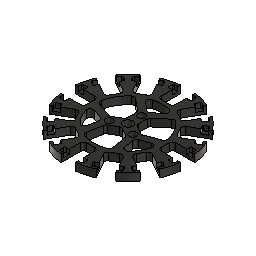
omni_wheel (Autodesk Fusion 360 archive; units mm, degrees)
design "omni_inside_world"
Autodesk Fusion 360 part; units mm, degrees
(part 1 of 2)
sketch "スケッチ1" plane through (0, 0, 0) normal (0, 0, 1) x (1, 0, 0)
  circle A0 centre (0, 0) radius 27.5
  line L0 (0, 0) -> (0, 27.5)
  line L1 (0, 27.5) -> (0, 17)
  line L2 (0, 17) -> (3.3, 17)
  line L3 (3.3, 17) -> (3.3, 27.3013)
  line L4 (3.3, 17) -> (-3.3, 17)
  line L5 (-3.3, 17) -> (-3.3, 27.5)
  line L6 (-3.3, 27.5) -> (3.3, 27.5)
  line L7 (3.3, 27.5) -> (3.3, 17)
  line L8 (-11.3579, 13.0724) -> (-16.6079, 22.1657)
  line L9 (-5.6421, 16.3724) -> (-11.3579, 13.0724)
  line L10 (-5.6421, 16.3724) -> (-10.7928, 25.2936)
  line L11 (-16.6079, 22.1657) -> (-10.8921, 25.4657)
  line L12 (-8.5, 14.7224) -> (-5.6421, 16.3724)
  line L13 (-16.3724, 5.6421) -> (-25.4657, 10.8921)
  line L14 (-13.0724, 11.3579) -> (-16.3724, 5.6421)
  line L15 (-13.0724, 11.3579) -> (-21.9936, 16.5085)
  line L16 (-25.4657, 10.8921) -> (-22.1657, 16.6079)
  line L17 (-14.7224, 8.5) -> (-13.0724, 11.3579)
  line L18 (-17, -3.3) -> (-27.5, -3.3)
  line L19 (-17, 3.3) -> (-17, -3.3)
  line L20 (-17, 3.3) -> (-27.3013, 3.3)
  line L21 (-27.5, -3.3) -> (-27.5, 3.3)
  line L22 (-17, 0) -> (-17, 3.3)
  line L23 (-13.0724, -11.3579) -> (-22.1657, -16.6079)
  line L24 (-16.3724, -5.6421) -> (-13.0724, -11.3579)
  line L25 (-16.3724, -5.6421) -> (-25.2936, -10.7928)
  line L26 (-22.1657, -16.6079) -> (-25.4657, -10.8921)
  line L27 (-14.7224, -8.5) -> (-16.3724, -5.6421)
  line L28 (-5.6421, -16.3724) -> (-10.8921, -25.4657)
  line L29 (-11.3579, -13.0724) -> (-5.6421, -16.3724)
  line L30 (-11.3579, -13.0724) -> (-16.5085, -21.9936)
  line L31 (-10.8921, -25.4657) -> (-16.6079, -22.1657)
  line L32 (-8.5, -14.7224) -> (-11.3579, -13.0724)
  line L33 (3.3, -17) -> (3.3, -27.5)
  line L34 (-3.3, -17) -> (3.3, -17)
  line L35 (-3.3, -17) -> (-3.3, -27.3013)
  line L36 (3.3, -27.5) -> (-3.3, -27.5)
  line L37 (0, -17) -> (-3.3, -17)
  line L38 (11.3579, -13.0724) -> (16.6079, -22.1657)
  line L39 (5.6421, -16.3724) -> (11.3579, -13.0724)
  line L40 (5.6421, -16.3724) -> (10.7928, -25.2936)
  line L41 (16.6079, -22.1657) -> (10.8921, -25.4657)
  line L42 (8.5, -14.7224) -> (5.6421, -16.3724)
  line L43 (16.3724, -5.6421) -> (25.4657, -10.8921)
  line L44 (13.0724, -11.3579) -> (16.3724, -5.6421)
  line L45 (13.0724, -11.3579) -> (21.9936, -16.5085)
  line L46 (25.4657, -10.8921) -> (22.1657, -16.6079)
  line L47 (14.7224, -8.5) -> (13.0724, -11.3579)
  line L48 (17, 3.3) -> (27.5, 3.3)
  line L49 (17, -3.3) -> (17, 3.3)
  line L50 (17, -3.3) -> (27.3013, -3.3)
  line L51 (27.5, 3.3) -> (27.5, -3.3)
  line L52 (17, 0) -> (17, -3.3)
  line L53 (13.0724, 11.3579) -> (22.1657, 16.6079)
  line L54 (16.3724, 5.6421) -> (13.0724, 11.3579)
  line L55 (16.3724, 5.6421) -> (25.2936, 10.7928)
  line L56 (22.1657, 16.6079) -> (25.4657, 10.8921)
  line L57 (14.7224, 8.5) -> (16.3724, 5.6421)
  line L58 (5.6421, 16.3724) -> (10.8921, 25.4657)
  line L59 (11.3579, 13.0724) -> (5.6421, 16.3724)
  line L60 (11.3579, 13.0724) -> (16.5085, 21.9936)
  line L61 (10.8921, 25.4657) -> (16.6079, 22.1657)
  line L62 (8.5, 14.7224) -> (11.3579, 13.0724)
  line L63 (0, 17) -> (0, 15.5)
  circle A1 centre (0, 0) radius 15.5
  circle A2 centre (0, 0) radius 2.1
  line L64 (0, 2.1) -> (2.5, 2.1)
  line L65 (2.5, 2.1) -> (2.5, 15.2971)
  line L66 (2.5, 2.1) -> (-2.5, 2.1)
  line L67 (-2.5, 2.1) -> (-2.5, 15.2971)
  line L68 (-2.5, 15.2971) -> (2.5, 15.2971)
  line L69 (2.5, 15.2971) -> (2.5, 2.1)
  line L70 (-2.5, 2.1) -> (2.5, 2.1)
  line L71 (2.5, 2.1) -> (2.5, 0)
  line L72 (2.5, 0) -> (-2.5, 0)
  line L73 (-2.5, 0) -> (-2.5, 2.1)
  line L74 (1.25, -2.1651) -> (-0.5687, -3.2151)
  line L75 (-0.5687, -3.2151) -> (-11.9976, -9.8136)
  line L76 (-3.0687, 1.1151) -> (-1.25, 2.1651)
  line L77 (-3.0687, 1.1151) -> (-14.4976, -5.4835)
  line L78 (-1.25, 2.1651) -> (1.25, -2.1651)
  line L79 (1.25, 2.1651) -> (3.0687, 1.1151)
  line L80 (3.0687, 1.1151) -> (14.4976, -5.4835)
  line L81 (0.5687, -3.2151) -> (-1.25, -2.1651)
  line L82 (0.5687, -3.2151) -> (11.9976, -9.8136)
  line L83 (-1.25, -2.1651) -> (1.25, 2.1651)
  line L84 (0, 0) -> (0, 6.8)
  line L85 (0, 6.8) -> (-2.5, 6.8)
  line L86 (0, 6.8) -> (2.5, 6.8)
  line L87 (0, 6.8) -> (7.8674, 13.3549)
  line L88 (0, 6.8) -> (9.0795, 6.8) construction
  line L89 (0, 6.8) -> (0.9602, 5.6476)
  line L90 (0.9602, 5.6476) -> (9.1755, 12.4924)
  line L91 (0, 6.8) -> (-0.9602, 7.9524)
  line L92 (-0.9602, 7.9524) -> (6.4251, 14.1056)
  line L93 (0.9602, 7.9524) -> (-6.4251, 14.1056)
  line L94 (-0.9602, 5.6476) -> (-9.1755, 12.4924)
  line L95 (0, 6.8) -> (-7.8674, 13.3549)
  line L96 (0, 6.8) -> (-0.9602, 5.6476)
  line L97 (0, 6.8) -> (0.9602, 7.9524)
  line L98 (-7.3671, -3.1447) -> (-9.0033, -12.6171)
  line L99 (-5.889, -3.4) -> (-7.632, -13.4909)
  line L100 (-4.4109, -3.6553) -> (-6.2309, -14.1924)
  line L101 (-6.4069, -4.8077) -> (-15.4284, -1.4885)
  line L102 (-5.889, -3.4) -> (-15.4994, 0.136)
  line L103 (-5.371, -1.9923) -> (-15.4065, 1.7001)
  line L104 (-5.889, -3.4) -> (-5.371, -1.9923)
  line L105 (-5.889, -3.4) -> (-4.4109, -3.6553)
  line L106 (-5.889, -3.4) -> (-6.4069, -4.8077)
  line L107 (-5.889, -3.4) -> (-7.3671, -3.1447)
  line L108 (6.4069, -4.8077) -> (15.4284, -1.4885)
  line L109 (5.889, -3.4) -> (15.4994, 0.136)
  line L110 (5.371, -1.9923) -> (15.4065, 1.7001)
  line L111 (7.3671, -3.1447) -> (9.0033, -12.6171)
  line L112 (5.889, -3.4) -> (7.632, -13.4909)
  line L113 (4.4109, -3.6553) -> (6.2309, -14.1924)
  line L114 (5.889, -3.4) -> (4.4109, -3.6553)
  line L115 (5.889, -3.4) -> (5.371, -1.9923)
  line L116 (5.889, -3.4) -> (7.3671, -3.1447)
  line L117 (5.889, -3.4) -> (6.4069, -4.8077)
  dimension "d1" = 55
  dimension "d2" = 10.5
  dimension "d3" = 3.3
  dimension "d4" = 6.6
  dimension "d5" = 10.5
  dimension "d7" = 360
  dimension "d8" = 1.5
  dimension "d9" = 4.2
  dimension "d10" = 2.5
  dimension "d11" = 5
  dimension "d12" = 5
  dimension "d13" = 2.1
  dimension "d15" = 360
  dimension "d16" = 6.8
  dimension "d17" = 39.8
  dimension "d18" = 1.5
  dimension "d19" = 1.5
  dimension "d56" = 360
  constraint coincident A0.centre L0.start
  constraint coincident A0 L0.end
  constraint vertical L0
  constraint parallel L0 L1
  constraint perpendicular L0 L2
  constraint coincident A0 L3.end
  constraint perpendicular L2 L3
  constraint horizontal L4
  constraint vertical L5
  constraint horizontal L6
  constraint vertical L7
  constraint perpendicular L2 L63
  constraint concentric A0 A1
  constraint coincident L63.end A1
  constraint coincident L0 L64.start
  constraint coincident A2 L64.start
  constraint perpendicular L0 L64
  constraint coincident A1 L65.end
  constraint perpendicular L64 L65
  constraint horizontal L66
  constraint vertical L67
  constraint horizontal L68
  constraint vertical L69
  constraint coincident A1 L67.end
  constraint horizontal L70
  constraint vertical L71
  constraint horizontal L72
  constraint vertical L73
  constraint parallel L0 L84
  constraint coincident L67 L85.end
  constraint perpendicular L67 L85
  constraint coincident L69 L86.end
  constraint perpendicular L69 L86
  constraint horizontal L88
  constraint coincident A1 L87.end
  constraint perpendicular L87 L89
  constraint coincident A1 L90.end
  constraint perpendicular L89 L90
  constraint perpendicular L87 L91
  constraint coincident A1 L92.end
  constraint perpendicular L91 L92
  constraint symmetric L0 L84.end L85.start
  constraint symmetric L0 L87.end L95.end
  constraint symmetric L0 L89.end L94.start
  constraint symmetric L0 L90.end L94.end
  constraint symmetric L0 L91.end L93.start
  constraint symmetric L0 L92.end L93.end
  measures "d1" diameter of A0
  measures "d2" distance of L0.end L1.end
  measures "d3" distance of L1.end L2.end
  measures "d4" distance of L2.end L4.end
  measures "d5" distance of L2.end L6.end
  measures "d8" distance of L1.end L63.end
  measures "d9" diameter of A2
  measures "d10" distance of L64.start L64.end
  measures "d11" distance of L64.end L66.end
  measures "d12" distance of L66.end L64.end
  measures "d13" distance of L66.end L72.end
  measures "d16" distance of A0.centre L84.end
  measures "d17" angle of L87 L88
  measures "d18" distance of L84.end L89.end
  measures "d19" distance of L84.end L91.end
extrude "押し出し1" add sketch "スケッチ1" along normal blind 1.5 contours A0 L2 L3 L4 L5 L7 L8 L9 L10 L12 L13 L14 L15 L17 L18 L19 L20 L22 L23 L24 L25 L27 L28 L29 L30 L32 L33 L34 L35 L37 L38 L39 L40 L42 L43 L44 L45 L47 L48 L49 L50 L52 L53 L54 L55 L57 L58 L59 L60 L62 | L0 L66 L67 L70 L76 L78 L84 L85 L94 L96 | A2 L64 L66 L70 L83 | L0 L64 L65 L66 L69 L70 L79 L83 L84 L86 L89 L90 | A2 L66 L70 L78 | A2 L71 L72 L74 L78 L79 L80 L81 L82 L110 L113 L114 L115 | A2 L64 L66 L70 L71 L72 L79 L83 | A2 L66 L70 L72 L73 L76 L78 | A2 L72 L73 L74 L75 L76 L77 L81 L83 L100 L103 L104 L105 | A2 L74 L78 L81 L83 | L0 L91 L92 | L85 L94 L96 | L65 L69 L86 L87 L90 | L65 L69 L87 L92 L93 L97 | L86 L89 L90 | L67 L91 L92 L93 L95 | L67 L85 L94 L95 | L0 L93 L97 | L64 L66 L70 L79 L83 | L66 L70 L76 L78 | L67 L85 L94 | L65 L69 L86 L90 | A1 L65 L69 L87 L90 | A1 L65 L69 L87 L92 | A1 L67 L93 L95 | A1 L67 L94 L95 | L64 L66 L70 L71 L79 | L66 L70 L73 L76 | A1 L80 L109 L110 | L80 L109 L110 L115 | L77 L102 L103 L104 | A1 L77 L102 L103 | A1 L75 L99 L100 | L75 L99 L100 L105 | L82 L112 L113 L114 | A1 L82 L112 L113 | A1 L80 L108 L109 | L80 L108 L109 L111 L116 | L77 L98 L101 L102 L107 | A1 L77 L101 L102 | A1 L75 L98 L99 | L75 L98 L99 L101 L106 | L82 L108 L111 L112 L117 | A1 L82 L111 L112 | L108 L111 L116 L117 | L98 L101 L106 L107
sketch "スケッチ2" plane through (0, 0, 1.5) normal (0, 0, 1) x (-1, 0, 0)
  line L0 (-5.6421, -16.3724) -> (-10.7928, -25.2936)
  arc A0 (-10.7928, -25.2936) -> (-3.3, -27.3013) centre (0, 0) ccw
  line L1 (-3.3, -27.3013) -> (-3.3, -17)
  line L2 (-3.3, -17) -> (3.3, -17)
  line L3 (3.3, -17) -> (3.3, -27.3013)
  arc A1 (3.3, -27.3013) -> (10.7928, -25.2936) centre (0, 0) ccw
  line L4 (10.7928, -25.2936) -> (5.6421, -16.3724)
  line L5 (5.6421, -16.3724) -> (11.3579, -13.0724)
  line L6 (11.3579, -13.0724) -> (16.5085, -21.9936)
  arc A2 (16.5085, -21.9936) -> (21.9936, -16.5085) centre (0, 0) ccw
  line L7 (21.9936, -16.5085) -> (13.0724, -11.3579)
  line L8 (13.0724, -11.3579) -> (16.3724, -5.6421)
  line L9 (16.3724, -5.6421) -> (25.2936, -10.7928)
  arc A3 (25.2936, -10.7928) -> (27.3013, -3.3) centre (0, 0) ccw
  line L10 (27.3013, -3.3) -> (17, -3.3)
  line L11 (17, -3.3) -> (17, 3.3)
  line L12 (17, 3.3) -> (27.3013, 3.3)
  arc A4 (27.3013, 3.3) -> (25.2936, 10.7928) centre (0, 0) ccw
  line L13 (25.2936, 10.7928) -> (16.3724, 5.6421)
  line L14 (16.3724, 5.6421) -> (13.0724, 11.3579)
  line L15 (13.0724, 11.3579) -> (21.9936, 16.5085)
  arc A5 (21.9936, 16.5085) -> (16.5085, 21.9936) centre (0, 0) ccw
  line L16 (16.5085, 21.9936) -> (11.3579, 13.0724)
  line L17 (11.3579, 13.0724) -> (5.6421, 16.3724)
  line L18 (5.6421, 16.3724) -> (10.7928, 25.2936)
  arc A6 (10.7928, 25.2936) -> (3.3, 27.3013) centre (0, 0) ccw
  line L19 (3.3, 27.3013) -> (3.3, 17)
  line L20 (3.3, 17) -> (-3.3, 17)
  line L21 (-3.3, 17) -> (-3.3, 27.3013)
  arc A7 (-3.3, 27.3013) -> (-10.7928, 25.2936) centre (0, 0) ccw
  line L22 (-10.7928, 25.2936) -> (-5.6421, 16.3724)
  line L23 (-5.6421, 16.3724) -> (-11.3579, 13.0724)
  line L24 (-11.3579, 13.0724) -> (-16.5085, 21.9936)
  arc A8 (-16.5085, 21.9936) -> (-21.9936, 16.5085) centre (0, 0) ccw
  line L25 (-21.9936, 16.5085) -> (-13.0724, 11.3579)
  line L26 (-13.0724, 11.3579) -> (-16.3724, 5.6421)
  line L27 (-16.3724, 5.6421) -> (-25.2936, 10.7928)
  arc A9 (-25.2936, 10.7928) -> (-27.3013, 3.3) centre (0, 0) ccw
  line L28 (-27.3013, 3.3) -> (-17, 3.3)
  line L29 (-17, 3.3) -> (-17, -3.3)
  line L30 (-17, -3.3) -> (-27.3013, -3.3)
  arc A10 (-27.3013, -3.3) -> (-25.2936, -10.7928) centre (0, 0) ccw
  line L31 (-25.2936, -10.7928) -> (-16.3724, -5.6421)
  line L32 (-16.3724, -5.6421) -> (-13.0724, -11.3579)
  line L33 (-13.0724, -11.3579) -> (-21.9936, -16.5085)
  arc A11 (-21.9936, -16.5085) -> (-16.5085, -21.9936) centre (0, 0) ccw
  line L34 (-16.5085, -21.9936) -> (-11.3579, -13.0724)
  line L35 (-11.3579, -13.0724) -> (-5.6421, -16.3724)
  line L36 (0, 0) -> (0, -6.25)
  circle A12 centre (0, -6.25) radius 2.5
  circle A13 centre (0, -6.25) radius 1.65
  circle A14 centre (5.4127, 3.125) radius 2.5
  circle A15 centre (5.4127, 3.125) radius 1.65
  circle A16 centre (-5.4127, 3.125) radius 2.5
  circle A17 centre (-5.4127, 3.125) radius 1.65
  line L37 (4.752, 5.6303) -> (0, 2.8868)
  line L38 (0, 2.8868) -> (-4.752, 5.6303)
  line L39 (-4.752, 5.6303) -> (-6.2309, 14.1924)
  arc A18 (6.2309, 14.1924) -> (-6.2309, 14.1924) centre (0, 0) ccw
  line L40 (6.2309, 14.1924) -> (4.752, 5.6303)
  circle A19 centre (0, 0) radius 2.1
  arc A20 (15.4284, 1.4885) -> (9.0033, 12.6171) centre (0, 0) ccw
  line L41 (15.4284, 1.4885) -> (7.5798, 4.3762)
  line L42 (7.5798, 4.3762) -> (9.0033, 12.6171)
  line L43 (2.5, -6.9305) -> (2.5, -1.4434)
  line L44 (2.5, -1.4434) -> (7.252, 1.3002)
  line L45 (7.252, 1.3002) -> (15.4065, -1.7001)
  arc A21 (9.1755, -12.4924) -> (15.4065, -1.7001) centre (0, 0) ccw
  line L46 (9.1755, -12.4924) -> (2.5, -6.9305)
  arc A22 (-9.0033, 12.6171) -> (-15.4284, 1.4885) centre (0, 0) ccw
  line L47 (-9.0033, 12.6171) -> (-7.5798, 4.3762)
  line L48 (-7.5798, 4.3762) -> (-15.4284, 1.4885)
  line L49 (-6.4251, -14.1056) -> (0, -8.7524)
  line L50 (0, -8.7524) -> (6.4251, -14.1056)
  arc A23 (-6.4251, -14.1056) -> (6.4251, -14.1056) centre (0, 0) ccw
  line L51 (-2.5, -6.9305) -> (-9.1755, -12.4924)
  arc A24 (-15.4065, -1.7001) -> (-9.1755, -12.4924) centre (0, 0) ccw
  line L52 (-15.4065, -1.7001) -> (-7.252, 1.3002)
  line L53 (-7.252, 1.3002) -> (-2.5, -1.4434)
  line L54 (-2.5, -1.4434) -> (-2.5, -6.9305)
  dimension "d25" = 6.25
  dimension "d26" = 5
  dimension "d27" = 3.3
  dimension "d29" = 360
  constraint coincident A0.centre A1.centre
  constraint vertical L36
  constraint coincident L36.end A12.centre
  constraint concentric A12 A13
  measures "d25" distance of A0.centre L36.end
  measures "d26" diameter of A12
  measures "d27" diameter of A13
extrude "押し出し2" cut sketch "スケッチ2" against normal blind 1.5 contours A13 | A15 | A17
sketch "スケッチ3" plane through (0, 0, 1.5) normal (0, 0, 1) x (-1, 0, 0)
  line L0 (-5.6421, -16.3724) -> (-10.7928, -25.2936)
  arc A0 (-10.7928, -25.2936) -> (-3.3, -27.3013) centre (0, 0) ccw
  line L1 (-3.3, -27.3013) -> (-3.3, -17)
  line L2 (-3.3, -17) -> (3.3, -17)
  line L3 (3.3, -17) -> (3.3, -27.3013)
  arc A1 (3.3, -27.3013) -> (10.7928, -25.2936) centre (0, 0) ccw
  line L4 (10.7928, -25.2936) -> (5.6421, -16.3724)
  line L5 (5.6421, -16.3724) -> (11.3579, -13.0724)
  line L6 (11.3579, -13.0724) -> (16.5085, -21.9936)
  arc A2 (16.5085, -21.9936) -> (21.9936, -16.5085) centre (0, 0) ccw
  line L7 (21.9936, -16.5085) -> (13.0724, -11.3579)
  line L8 (13.0724, -11.3579) -> (16.3724, -5.6421)
  line L9 (16.3724, -5.6421) -> (25.2936, -10.7928)
  arc A3 (25.2936, -10.7928) -> (27.3013, -3.3) centre (0, 0) ccw
  line L10 (27.3013, -3.3) -> (17, -3.3)
  line L11 (17, -3.3) -> (17, 3.3)
  line L12 (17, 3.3) -> (27.3013, 3.3)
  arc A4 (27.3013, 3.3) -> (25.2936, 10.7928) centre (0, 0) ccw
  line L13 (25.2936, 10.7928) -> (16.3724, 5.6421)
  line L14 (16.3724, 5.6421) -> (13.0724, 11.3579)
  line L15 (13.0724, 11.3579) -> (21.9936, 16.5085)
  arc A5 (21.9936, 16.5085) -> (16.5085, 21.9936) centre (0, 0) ccw
  line L16 (16.5085, 21.9936) -> (11.3579, 13.0724)
  line L17 (11.3579, 13.0724) -> (5.6421, 16.3724)
  line L18 (5.6421, 16.3724) -> (10.7928, 25.2936)
  arc A6 (10.7928, 25.2936) -> (3.3, 27.3013) centre (0, 0) ccw
  line L19 (3.3, 27.3013) -> (3.3, 17)
  line L20 (3.3, 17) -> (-3.3, 17)
  line L21 (-3.3, 17) -> (-3.3, 27.3013)
  arc A7 (-3.3, 27.3013) -> (-10.7928, 25.2936) centre (0, 0) ccw
  line L22 (-10.7928, 25.2936) -> (-5.6421, 16.3724)
  line L23 (-5.6421, 16.3724) -> (-11.3579, 13.0724)
  line L24 (-11.3579, 13.0724) -> (-16.5085, 21.9936)
  arc A8 (-16.5085, 21.9936) -> (-21.9936, 16.5085) centre (0, 0) ccw
  line L25 (-21.9936, 16.5085) -> (-13.0724, 11.3579)
  line L26 (-13.0724, 11.3579) -> (-16.3724, 5.6421)
  line L27 (-16.3724, 5.6421) -> (-25.2936, 10.7928)
  arc A9 (-25.2936, 10.7928) -> (-27.3013, 3.3) centre (0, 0) ccw
  line L28 (-27.3013, 3.3) -> (-17, 3.3)
  line L29 (-17, 3.3) -> (-17, -3.3)
  line L30 (-17, -3.3) -> (-27.3013, -3.3)
  arc A10 (-27.3013, -3.3) -> (-25.2936, -10.7928) centre (0, 0) ccw
  line L31 (-25.2936, -10.7928) -> (-16.3724, -5.6421)
  line L32 (-16.3724, -5.6421) -> (-13.0724, -11.3579)
  line L33 (-13.0724, -11.3579) -> (-21.9936, -16.5085)
  arc A11 (-21.9936, -16.5085) -> (-16.5085, -21.9936) centre (0, 0) ccw
  line L34 (-16.5085, -21.9936) -> (-11.3579, -13.0724)
  line L35 (-11.3579, -13.0724) -> (-5.6421, -16.3724)
  line L36 (3.3, -27.3013) -> (3.3, -26.1013)
  line L37 (3.3, -26.1013) -> (3.3, -23.5013)
  line L38 (3.3, -23.5013) -> (5.3, -23.5013)
  line L39 (5.3, -23.5013) -> (5.3, -26.1013)
  line L40 (5.3, -26.1013) -> (3.3, -26.1013)
  line L41 (3.3, -26.1013) -> (3.3, -23.5013)
  line L42 (-3.3, -27.3013) -> (-3.3, -26.1013)
  line L43 (-3.3, -26.1013) -> (-5.3, -26.1013)
  line L44 (-5.3, -26.1013) -> (-5.3, -23.5013)
  line L45 (-5.3, -23.5013) -> (-3.3, -23.5013)
  line L46 (-3.3, -23.5013) -> (-3.3, -26.1013)
  line L47 (14.6085, -18.7027) -> (16.3406, -17.7027)
  line L48 (16.3406, -17.7027) -> (17.6406, -19.9544)
  line L49 (17.6406, -19.9544) -> (15.9085, -20.9544)
  line L50 (15.9085, -20.9544) -> (14.6085, -18.7027)
  line L51 (8.8928, -22.0027) -> (10.1928, -24.2544)
  line L52 (7.1607, -23.0027) -> (8.8928, -22.0027)
  line L53 (8.4607, -25.2544) -> (7.1607, -23.0027)
  line L54 (10.1928, -24.2544) -> (8.4607, -25.2544)
  line L55 (22.0027, -8.8928) -> (23.0027, -7.1607)
  line L56 (23.0027, -7.1607) -> (25.2544, -8.4607)
  line L57 (25.2544, -8.4607) -> (24.2544, -10.1928)
  line L58 (24.2544, -10.1928) -> (22.0027, -8.8928)
  line L59 (18.7027, -14.6085) -> (20.9544, -15.9085)
  line L60 (17.7027, -16.3406) -> (18.7027, -14.6085)
  line L61 (19.9544, -17.6406) -> (17.7027, -16.3406)
  line L62 (20.9544, -15.9085) -> (19.9544, -17.6406)
  line L63 (23.5013, 3.3) -> (23.5013, 5.3)
  line L64 (23.5013, 5.3) -> (26.1013, 5.3)
  line L65 (26.1013, 5.3) -> (26.1013, 3.3)
  line L66 (26.1013, 3.3) -> (23.5013, 3.3)
  line L67 (23.5013, -3.3) -> (26.1013, -3.3)
  line L68 (23.5013, -5.3) -> (23.5013, -3.3)
  line L69 (26.1013, -5.3) -> (23.5013, -5.3)
  line L70 (26.1013, -3.3) -> (26.1013, -5.3)
  line L71 (18.7027, 14.6085) -> (17.7027, 16.3406)
  line L72 (17.7027, 16.3406) -> (19.9544, 17.6406)
  line L73 (19.9544, 17.6406) -> (20.9544, 15.9085)
  line L74 (20.9544, 15.9085) -> (18.7027, 14.6085)
  line L75 (22.0027, 8.8928) -> (24.2544, 10.1928)
  line L76 (23.0027, 7.1607) -> (22.0027, 8.8928)
  line L77 (25.2544, 8.4607) -> (23.0027, 7.1607)
  line L78 (24.2544, 10.1928) -> (25.2544, 8.4607)
  line L79 (8.8928, 22.0027) -> (7.1607, 23.0027)
  line L80 (7.1607, 23.0027) -> (8.4607, 25.2544)
  line L81 (8.4607, 25.2544) -> (10.1928, 24.2544)
  line L82 (10.1928, 24.2544) -> (8.8928, 22.0027)
  line L83 (14.6085, 18.7027) -> (15.9085, 20.9544)
  line L84 (16.3406, 17.7027) -> (14.6085, 18.7027)
  line L85 (17.6406, 19.9544) -> (16.3406, 17.7027)
  line L86 (15.9085, 20.9544) -> (17.6406, 19.9544)
  line L87 (-3.3, 23.5013) -> (-5.3, 23.5013)
  line L88 (-5.3, 23.5013) -> (-5.3, 26.1013)
  line L89 (-5.3, 26.1013) -> (-3.3, 26.1013)
  line L90 (-3.3, 26.1013) -> (-3.3, 23.5013)
  line L91 (3.3, 23.5013) -> (3.3, 26.1013)
  line L92 (5.3, 23.5013) -> (3.3, 23.5013)
  line L93 (5.3, 26.1013) -> (5.3, 23.5013)
  line L94 (3.3, 26.1013) -> (5.3, 26.1013)
  line L95 (-14.6085, 18.7027) -> (-16.3406, 17.7027)
  line L96 (-16.3406, 17.7027) -> (-17.6406, 19.9544)
  line L97 (-17.6406, 19.9544) -> (-15.9085, 20.9544)
  line L98 (-15.9085, 20.9544) -> (-14.6085, 18.7027)
  line L99 (-8.8928, 22.0027) -> (-10.1928, 24.2544)
  line L100 (-7.1607, 23.0027) -> (-8.8928, 22.0027)
  line L101 (-8.4607, 25.2544) -> (-7.1607, 23.0027)
  line L102 (-10.1928, 24.2544) -> (-8.4607, 25.2544)
  line L103 (-22.0027, 8.8928) -> (-23.0027, 7.1607)
  line L104 (-23.0027, 7.1607) -> (-25.2544, 8.4607)
  line L105 (-25.2544, 8.4607) -> (-24.2544, 10.1928)
  line L106 (-24.2544, 10.1928) -> (-22.0027, 8.8928)
  line L107 (-18.7027, 14.6085) -> (-20.9544, 15.9085)
  line L108 (-17.7027, 16.3406) -> (-18.7027, 14.6085)
  line L109 (-19.9544, 17.6406) -> (-17.7027, 16.3406)
  line L110 (-20.9544, 15.9085) -> (-19.9544, 17.6406)
  line L111 (-23.5013, -3.3) -> (-23.5013, -5.3)
  line L112 (-23.5013, -5.3) -> (-26.1013, -5.3)
  line L113 (-26.1013, -5.3) -> (-26.1013, -3.3)
  line L114 (-26.1013, -3.3) -> (-23.5013, -3.3)
  line L115 (-23.5013, 3.3) -> (-26.1013, 3.3)
  line L116 (-23.5013, 5.3) -> (-23.5013, 3.3)
  line L117 (-26.1013, 5.3) -> (-23.5013, 5.3)
  line L118 (-26.1013, 3.3) -> (-26.1013, 5.3)
  line L119 (-18.7027, -14.6085) -> (-17.7027, -16.3406)
  line L120 (-17.7027, -16.3406) -> (-19.9544, -17.6406)
  line L121 (-19.9544, -17.6406) -> (-20.9544, -15.9085)
  line L122 (-20.9544, -15.9085) -> (-18.7027, -14.6085)
  line L123 (-22.0027, -8.8928) -> (-24.2544, -10.1928)
  line L124 (-23.0027, -7.1607) -> (-22.0027, -8.8928)
  line L125 (-25.2544, -8.4607) -> (-23.0027, -7.1607)
  line L126 (-24.2544, -10.1928) -> (-25.2544, -8.4607)
  line L127 (-8.8928, -22.0027) -> (-7.1607, -23.0027)
  line L128 (-7.1607, -23.0027) -> (-8.4607, -25.2544)
  line L129 (-8.4607, -25.2544) -> (-10.1928, -24.2544)
  line L130 (-10.1928, -24.2544) -> (-8.8928, -22.0027)
  line L131 (-14.6085, -18.7027) -> (-15.9085, -20.9544)
  line L132 (-16.3406, -17.7027) -> (-14.6085, -18.7027)
  line L133 (-17.6406, -19.9544) -> (-16.3406, -17.7027)
  line L134 (-15.9085, -20.9544) -> (-17.6406, -19.9544)
  circle A12 centre (0, -6.25) radius 1.65
  circle A13 centre (5.4127, 3.125) radius 1.65
  circle A14 centre (-5.4127, 3.125) radius 1.65
  line L135 (4.752, 5.6303) -> (0, 2.8868)
  line L136 (0, 2.8868) -> (-4.752, 5.6303)
  line L137 (-4.752, 5.6303) -> (-6.2309, 14.1924)
  arc A15 (6.2309, 14.1924) -> (-6.2309, 14.1924) centre (0, 0) ccw
  line L138 (6.2309, 14.1924) -> (4.752, 5.6303)
  circle A16 centre (0, 0) radius 2.1
  arc A17 (15.4284, 1.4885) -> (9.0033, 12.6171) centre (0, 0) ccw
  line L139 (15.4284, 1.4885) -> (7.5798, 4.3762)
  line L140 (7.5798, 4.3762) -> (9.0033, 12.6171)
  line L141 (2.5, -6.9305) -> (2.5, -1.4434)
  line L142 (2.5, -1.4434) -> (7.252, 1.3002)
  line L143 (7.252, 1.3002) -> (15.4065, -1.7001)
  arc A18 (9.1755, -12.4924) -> (15.4065, -1.7001) centre (0, 0) ccw
  line L144 (9.1755, -12.4924) -> (2.5, -6.9305)
  arc A19 (-9.0033, 12.6171) -> (-15.4284, 1.4885) centre (0, 0) ccw
  line L145 (-9.0033, 12.6171) -> (-7.5798, 4.3762)
  line L146 (-7.5798, 4.3762) -> (-15.4284, 1.4885)
  line L147 (-6.4251, -14.1056) -> (0, -8.7524)
  line L148 (0, -8.7524) -> (6.4251, -14.1056)
  arc A20 (-6.4251, -14.1056) -> (6.4251, -14.1056) centre (0, 0) ccw
  line L149 (-2.5, -6.9305) -> (-9.1755, -12.4924)
  arc A21 (-15.4065, -1.7001) -> (-9.1755, -12.4924) centre (0, 0) ccw
  line L150 (-15.4065, -1.7001) -> (-7.252, 1.3002)
  line L151 (-7.252, 1.3002) -> (-2.5, -1.4434)
  line L152 (-2.5, -1.4434) -> (-2.5, -6.9305)
  dimension "d32" = 1.2
  dimension "d33" = 2.6
  dimension "d34" = 2
  dimension "d35" = 2.6
  dimension "d36" = 1.2
  dimension "d37" = 2
  dimension "d38" = 2.6
  dimension "d40" = 360
  constraint coincident L3.end A1.start
  constraint vertical L36
  constraint parallel L3 L37
  constraint horizontal L38
  constraint vertical L39
  constraint horizontal L40
  constraint vertical L41
  constraint coincident A0.end L1.start
  constraint parallel L1 L42
  constraint horizontal L43
  constraint vertical L44
  constraint horizontal L45
  constraint vertical L46
  measures "d32" distance of L3.end L36.end
  measures "d33" distance of L36.end L37.end
  measures "d34" distance of L37.end L38.end
  measures "d35" distance of L37.end L36.end
  measures "d36" distance of A0.end L42.end
  measures "d37" distance of L42.end L43.end
  measures "d38" distance of L42.end L45.end
extrude "押し出し3" add sketch "スケッチ3" along normal blind 0.5 contours L0 A0 L1 L2 L3 A1 L4 L5 L6 A2 L7 L8 L9 A3 L10 L11 L12 A4 L13 L14 L15 A5 L16 L17 L18 A6 L19 L20 L21 A7 L22 L23 L24 A8 L25 L26 L27 A9 L28 L29 L30 A10 L31 L32 L33 A11 L34 L35 L36 L38 L39 L40 L42 L43 L44 L45 L47 L48 L49 L52 L53 L54 L55 L56 L57 L60 L61 L62 L63 L64 L65 L68 L69 L70 L71 L72 L73 L76 L77 L78 L79 L80 L81 L84 L85 L86 L87 L88 L89 L92 L93 L94 L95 L96 L97 L100 L101 L102 L103 L104 L105 L108 L109 L110 L111 L112 L113 L116 L117 L118 L119 L120 L121 L124 L125 L126 L127 L128 L129 L132 L133 L134
extrude "押し出し4" cut 1 faces at (12.6956, -0.3629, 0) along direction (0, 0, 1) blind 0.5
fillet "フィレット1" radius 1.5 10 edges at (-9.1755, 12.4924, 1.25) (0, -2.8868, 1.25) (-2.5, 1.4434, 1.25) (-2.5, 6.9305, 1.25) (0, 8.7524, 1.25) (-6.4251, 14.1056, 1.25) (6.4251, 14.1056, 1.25) (9.1755, 12.4924, 1.25) (2.5, 6.9305, 1.25) (2.5, 1.4434, 1.25)
fillet "フィレット1" radius 1.5 14 edges at (-4.752, -5.6303, 1.25) (-7.5798, -4.3762, 1.25) (-7.252, -1.3002, 1.25) (-15.4284, -1.4885, 1.25) (-15.4065, 1.7001, 1.25) (-6.2309, -14.1924, 1.25) (-9.0033, -12.6171, 1.25) (6.2309, -14.1924, 1.25) (9.0033, -12.6171, 1.25) (4.752, -5.6303, 1.25) (15.4284, -1.4885, 1.25) (7.5798, -4.3762, 1.25) (7.252, -1.3002, 1.25) (15.4065, 1.7001, 1.25)
fillet "フィレット2" radius 0.5 4 edges at (17.7027, 16.3406, 1.75) (19.9544, 17.6406, 1.75) (23.0027, 7.1607, 1.75) (25.2544, 8.4607, 1.75)
fillet "フィレット3" radius 0.5 44 edges at (17.6406, 19.9544, 1.75) (16.3406, 17.7027, 1.75) (8.4607, 25.2544, 1.75) (5.3, 23.5013, 1.75) (7.1607, 23.0027, 1.75) (5.3, 26.1013, 1.75) (-5.3, 23.5013, 1.75) (-5.3, 26.1013, 1.75) (-8.4607, 25.2544, 1.75) (-7.1607, 23.0027, 1.75) (-17.6406, 19.9544, 1.75) (-16.3406, 17.7027, 1.75) (-19.9544, 17.6406, 1.75) (-17.7027, 16.3406, 1.75) (-25.2544, 8.4607, 1.75) (-23.0027, 7.1607, 1.75) (-23.5013, 5.3, 1.75) (-26.1013, 5.3, 1.75) (-26.1013, -5.3, 1.75) (-23.5013, -5.3, 1.75) (-23.0027, -7.1607, 1.75) (-25.2544, -8.4607, 1.75) (-17.7027, -16.3406, 1.75) (-16.3406, -17.7027, 1.75) (-19.9544, -17.6406, 1.75) (-17.6406, -19.9544, 1.75) (-7.1607, -23.0027, 1.75) (-5.3, -23.5013, 1.75) (-5.3, -26.1013, 1.75) (-8.4607, -25.2544, 1.75) (7.1607, -23.0027, 1.75) (5.3, -23.5013, 1.75) (8.4607, -25.2544, 1.75) (5.3, -26.1013, 1.75) (16.3406, -17.7027, 1.75) (17.7027, -16.3406, 1.75) (19.9544, -17.6406, 1.75) (17.6406, -19.9544, 1.75) (23.5013, -5.3, 1.75) (23.0027, -7.1607, 1.75) (25.2544, -8.4607, 1.75) (26.1013, -5.3, 1.75) (26.1013, 5.3, 1.75) (23.5013, 5.3, 1.75)
fillet "フィレット4" radius 1.5 24 edges at (13.0724, 11.3579, 1.25) (11.3579, 13.0724, 1.25) (5.6421, 16.3724, 1.25) (3.3, 17, 1.25) (-3.3, 17, 1.25) (-5.6421, 16.3724, 1.25) (-11.3579, 13.0724, 1.25) (-13.0724, 11.3579, 1.25) (-16.3724, 5.6421, 1.25) (-17, 3.3, 1.25) (-17, -3.3, 1.25) (-16.3724, -5.6421, 1.25) (-13.0724, -11.3579, 1.25) (-11.3579, -13.0724, 1.25) (-5.6421, -16.3724, 1.25) (-3.3, -17, 1.25) (3.3, -17, 1.25) (5.6421, -16.3724, 1.25) (13.0724, -11.3579, 1.25) (11.3579, -13.0724, 1.25) (17, -3.3, 1.25) (16.3724, -5.6421, 1.25) (17, 3.3, 1.25) (16.3724, 5.6421, 1.25)
extrude "押し出し21" add 1 faces at (6.483, -9.7763, 2) along direction (0, 0, 1) blind 2
extrude "押し出し23" add 24 faces at (-19.7261, -15.9692, 1.5) (-15.9692, -19.7261, 1.5) (-8.8321, -23.2309, 1.5) (-3.9667, -24.5346, 1.5) (3.9667, -24.5346, 1.5) (8.8321, -23.2309, 1.5) (15.9692, -19.7261, 1.5) (19.7261, -15.9692, 1.5) (23.2309, -8.8321, 1.5) (24.5346, -3.9667, 1.5) (24.5346, 3.9667, 1.5) (23.6928, 9.0987, 1.5) (19.7261, 15.9692, 1.5) (15.9692, 19.7261, 1.5) (9.0987, 23.6928, 1.5) (3.9667, 25.0679, 1.5) (-3.9667, 24.5346, 1.5) (-9.0987, 23.6928, 1.5) (-15.9692, 19.7261, 1.5) (-19.7261, 15.9692, 1.5) (-23.6928, 9.0987, 1.5) (-25.0679, 3.9667, 1.5) (-24.5346, -3.9667, 1.5) (-23.6928, -9.0987, 1.5) along direction (0, 0, 1) blind 0.4

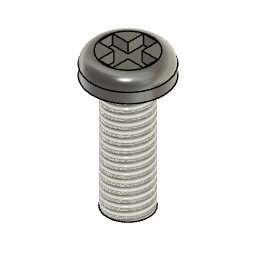
design "M3_8mm"
Autodesk Fusion 360 part; units mm, degrees
sketch "スケッチ1" plane through (0, 0, 0) normal (0, 0, 1) x (1, 0, 0)
  circle A0 centre (0, 0) radius 2.5
  circle A1 centre (0, 0) radius 1.5
  dimension "d1" = 5
  dimension "d2" = 3
  constraint coincident A0.centre A1.centre
  measures "d1" diameter of A0
  measures "d2" diameter of A1
extrude "押し出し1" add sketch "スケッチ1" along normal blind 1.5
sketch "スケッチ2" plane through (0, 0, 1.5) normal (0, 0, 1) x (-1, 0, 0)
  circle A0 centre (0, 0) radius 1.5
  circle A1 centre (0, 0) radius 2.5
  circle A2 centre (0, 0) radius 1.5
  constraint coincident A0.centre A1.centre
extrude "押し出し2" add sketch "スケッチ2" against normal blind 9.5 contours A0 A2
sketch "スケッチ3" plane through (0, 0, 1.5) normal (0, 0, 1) x (-1, 0, 0)
  circle A0 centre (0, 0) radius 2.5
  line L0 (0, 0) -> (0, -1.6)
  line L1 (0, -1.6) -> (0, 1.6)
  line L2 (0, 0) -> (-1.6, 0)
  line L3 (-1.6, 0) -> (1.6, 0)
  line L4 (0, 0) -> (0.5, 0)
  line L5 (0.5, 0) -> (0.5, -1.6)
  line L6 (0.5, -1.6) -> (0, -1.6)
  line L7 (0, -1.6) -> (0, 0)
  line L8 (0.5, -1.6) -> (-0.5, -1.6)
  line L9 (-0.5, -1.6) -> (-0.5, 1.6)
  line L10 (-0.5, 1.6) -> (0.5, 1.6)
  line L11 (0.5, 1.6) -> (0.5, -1.6)
  line L12 (1.6, 0) -> (-1.6, 0)
  line L13 (-1.6, 0) -> (-1.6, -0.5)
  line L14 (-1.6, -0.5) -> (1.6, -0.5)
  line L15 (1.6, -0.5) -> (1.6, 0)
  line L16 (-1.6, -0.5) -> (1.6, -0.5)
  line L17 (1.6, -0.5) -> (1.6, 0)
  line L18 (1.6, 0) -> (-1.6, 0)
  line L19 (-1.6, 0) -> (-1.6, -0.5)
  line L20 (-1.6, -0.5) -> (1.6, -0.5)
  line L21 (1.6, -0.5) -> (1.6, 0.5)
  line L22 (1.6, 0.5) -> (-1.6, 0.5)
  line L23 (-1.6, 0.5) -> (-1.6, -0.5)
  dimension "d7" = 1.6
  dimension "d8" = 3.2
  dimension "d9" = 1.6
  dimension "d10" = 3.2
  dimension "d11" = 0.5
  dimension "d12" = 1.6
  dimension "d13" = 1
  dimension "d14" = 0.5
  dimension "d15" = 0.5
  dimension "d16" = 1
  constraint coincident A0.centre L0.start
  constraint vertical L0
  constraint parallel L0 L1
  constraint perpendicular L0 L2
  constraint perpendicular L1 L3
  constraint horizontal L4
  constraint vertical L5
  constraint horizontal L6
  constraint vertical L7
  constraint horizontal L8
  constraint vertical L9
  constraint horizontal L10
  constraint vertical L11
  constraint horizontal L12
  constraint vertical L13
  constraint horizontal L14
  constraint vertical L15
  constraint horizontal L16
  constraint vertical L17
  constraint horizontal L18
  constraint vertical L19
  constraint horizontal L20
  constraint vertical L21
  constraint horizontal L22
  constraint vertical L23
  measures "d7" distance of A0.centre L0.end
  measures "d8" distance of L0.end L1.end
  measures "d9" distance of A0.centre L2.end
  measures "d10" distance of L2.end L3.end
  measures "d11" distance of A0.centre L4.end
  measures "d12" distance of A0.centre L0.end
  measures "d13" distance of L5.end L8.end
  measures "d14" distance of L3.end L14.end
  measures "d15" distance of L13.end L2.end
  measures "d16" distance of L13.end L22.end
extrude "押し出し3" cut sketch "スケッチ3" against normal blind 0.7 contours L0 L1 L3 L4 L5 L7 L11 L12 L14 L16 L18 L20 | L1 L2 L3 L9 L12 L18 L22 | L0 L1 L2 L3 L7 L9 L12 L14 L16 L18 L20 | L1 L3 L4 L11 L12 L18 L22 | L0 L1 L5 L6 L7 L8 L11 L14 L16 L20 | L0 L1 L7 L8 L9 L14 L16 L20 | L1 L9 L10 L22 | L1 L10 L11 L22 | L2 L3 L9 L12 L13 L14 L16 L18 L19 L20 L23 | L2 L3 L9 L12 L18 L22 L23 | L3 L11 L12 L18 L21 L22 | L3 L5 L11 L12 L14 L15 L16 L17 L18 L20 L21
fillet "フィレット1" radius 0.8 1 edges at (-2.3308, -0.904, 1.5)
thread "ねじ1" "ISO Metric profile 3.0 M3x0.5 6g" major diameter 2.927 minor diameter 2.3555 pitch 0.5 angle 60 resizes the face on face at (-1.4981, 0.0748, -5.3333)

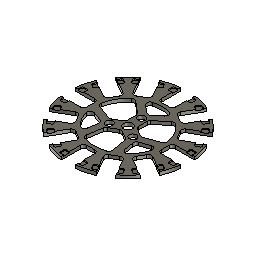
design "omni_outside_world"
Autodesk Fusion 360 part; units mm, degrees
sketch "スケッチ1" plane through (0, 0, 0) normal (0, 0, 1) x (1, 0, 0)
  circle A0 centre (0, 0) radius 27.5
  line L0 (0, 0) -> (0, 27.5)
  line L1 (0, 27.5) -> (0, 17)
  line L2 (0, 17) -> (3.3, 17)
  line L3 (3.3, 17) -> (3.3, 27.3013)
  line L4 (3.3, 17) -> (-3.3, 17)
  line L5 (-3.3, 17) -> (-3.3, 27.5)
  line L6 (-3.3, 27.5) -> (3.3, 27.5)
  line L7 (3.3, 27.5) -> (3.3, 17)
  line L8 (-11.3579, 13.0724) -> (-16.6079, 22.1657)
  line L9 (-5.6421, 16.3724) -> (-11.3579, 13.0724)
  line L10 (-5.6421, 16.3724) -> (-10.7928, 25.2936)
  line L11 (-16.6079, 22.1657) -> (-10.8921, 25.4657)
  line L12 (-8.5, 14.7224) -> (-5.6421, 16.3724)
  line L13 (-16.3724, 5.6421) -> (-25.4657, 10.8921)
  line L14 (-13.0724, 11.3579) -> (-16.3724, 5.6421)
  line L15 (-13.0724, 11.3579) -> (-21.9936, 16.5085)
  line L16 (-25.4657, 10.8921) -> (-22.1657, 16.6079)
  line L17 (-14.7224, 8.5) -> (-13.0724, 11.3579)
  line L18 (-17, -3.3) -> (-27.5, -3.3)
  line L19 (-17, 3.3) -> (-17, -3.3)
  line L20 (-17, 3.3) -> (-27.3013, 3.3)
  line L21 (-27.5, -3.3) -> (-27.5, 3.3)
  line L22 (-17, 0) -> (-17, 3.3)
  line L23 (-13.0724, -11.3579) -> (-22.1657, -16.6079)
  line L24 (-16.3724, -5.6421) -> (-13.0724, -11.3579)
  line L25 (-16.3724, -5.6421) -> (-25.2936, -10.7928)
  line L26 (-22.1657, -16.6079) -> (-25.4657, -10.8921)
  line L27 (-14.7224, -8.5) -> (-16.3724, -5.6421)
  line L28 (-5.6421, -16.3724) -> (-10.8921, -25.4657)
  line L29 (-11.3579, -13.0724) -> (-5.6421, -16.3724)
  line L30 (-11.3579, -13.0724) -> (-16.5085, -21.9936)
  line L31 (-10.8921, -25.4657) -> (-16.6079, -22.1657)
  line L32 (-8.5, -14.7224) -> (-11.3579, -13.0724)
  line L33 (3.3, -17) -> (3.3, -27.5)
  line L34 (-3.3, -17) -> (3.3, -17)
  line L35 (-3.3, -17) -> (-3.3, -27.3013)
  line L36 (3.3, -27.5) -> (-3.3, -27.5)
  line L37 (0, -17) -> (-3.3, -17)
  line L38 (11.3579, -13.0724) -> (16.6079, -22.1657)
  line L39 (5.6421, -16.3724) -> (11.3579, -13.0724)
  line L40 (5.6421, -16.3724) -> (10.7928, -25.2936)
  line L41 (16.6079, -22.1657) -> (10.8921, -25.4657)
  line L42 (8.5, -14.7224) -> (5.6421, -16.3724)
  line L43 (16.3724, -5.6421) -> (25.4657, -10.8921)
  line L44 (13.0724, -11.3579) -> (16.3724, -5.6421)
  line L45 (13.0724, -11.3579) -> (21.9936, -16.5085)
  line L46 (25.4657, -10.8921) -> (22.1657, -16.6079)
  line L47 (14.7224, -8.5) -> (13.0724, -11.3579)
  line L48 (17, 3.3) -> (27.5, 3.3)
  line L49 (17, -3.3) -> (17, 3.3)
  line L50 (17, -3.3) -> (27.3013, -3.3)
  line L51 (27.5, 3.3) -> (27.5, -3.3)
  line L52 (17, 0) -> (17, -3.3)
  line L53 (13.0724, 11.3579) -> (22.1657, 16.6079)
  line L54 (16.3724, 5.6421) -> (13.0724, 11.3579)
  line L55 (16.3724, 5.6421) -> (25.2936, 10.7928)
  line L56 (22.1657, 16.6079) -> (25.4657, 10.8921)
  line L57 (14.7224, 8.5) -> (16.3724, 5.6421)
  line L58 (5.6421, 16.3724) -> (10.8921, 25.4657)
  line L59 (11.3579, 13.0724) -> (5.6421, 16.3724)
  line L60 (11.3579, 13.0724) -> (16.5085, 21.9936)
  line L61 (10.8921, 25.4657) -> (16.6079, 22.1657)
  line L62 (8.5, 14.7224) -> (11.3579, 13.0724)
  line L63 (0, 17) -> (0, 15.5)
  circle A1 centre (0, 0) radius 15.5
  circle A2 centre (0, 0) radius 2.1
  line L64 (0, 2.1) -> (2.5, 2.1)
  line L65 (2.5, 2.1) -> (2.5, 15.2971)
  line L66 (2.5, 2.1) -> (-2.5, 2.1)
  line L67 (-2.5, 2.1) -> (-2.5, 15.2971)
  line L68 (-2.5, 15.2971) -> (2.5, 15.2971)
  line L69 (2.5, 15.2971) -> (2.5, 2.1)
  line L70 (-2.5, 2.1) -> (2.5, 2.1)
  line L71 (2.5, 2.1) -> (2.5, 0)
  line L72 (2.5, 0) -> (-2.5, 0)
  line L73 (-2.5, 0) -> (-2.5, 2.1)
  line L74 (1.25, -2.1651) -> (-0.5687, -3.2151)
  line L75 (-0.5687, -3.2151) -> (-11.9976, -9.8136)
  line L76 (-3.0687, 1.1151) -> (-1.25, 2.1651)
  line L77 (-3.0687, 1.1151) -> (-14.4976, -5.4835)
  line L78 (-1.25, 2.1651) -> (1.25, -2.1651)
  line L79 (1.25, 2.1651) -> (3.0687, 1.1151)
  line L80 (3.0687, 1.1151) -> (14.4976, -5.4835)
  line L81 (0.5687, -3.2151) -> (-1.25, -2.1651)
  line L82 (0.5687, -3.2151) -> (11.9976, -9.8136)
  line L83 (-1.25, -2.1651) -> (1.25, 2.1651)
  line L84 (0, 0) -> (0, 6.8)
  line L85 (0, 6.8) -> (-2.5, 6.8)
  line L86 (0, 6.8) -> (2.5, 6.8)
  line L87 (0, 6.8) -> (7.8674, 13.3549)
  line L88 (0, 6.8) -> (9.0795, 6.8) construction
  line L89 (0, 6.8) -> (0.9602, 5.6476)
  line L90 (0.9602, 5.6476) -> (9.1755, 12.4924)
  line L91 (0, 6.8) -> (-0.9602, 7.9524)
  line L92 (-0.9602, 7.9524) -> (6.4251, 14.1056)
  line L93 (0.9602, 7.9524) -> (-6.4251, 14.1056)
  line L94 (-0.9602, 5.6476) -> (-9.1755, 12.4924)
  line L95 (0, 6.8) -> (-7.8674, 13.3549)
  line L96 (0, 6.8) -> (-0.9602, 5.6476)
  line L97 (0, 6.8) -> (0.9602, 7.9524)
  line L98 (-7.3671, -3.1447) -> (-9.0033, -12.6171)
  line L99 (-5.889, -3.4) -> (-7.632, -13.4909)
  line L100 (-4.4109, -3.6553) -> (-6.2309, -14.1924)
  line L101 (-6.4069, -4.8077) -> (-15.4284, -1.4885)
  line L102 (-5.889, -3.4) -> (-15.4994, 0.136)
  line L103 (-5.371, -1.9923) -> (-15.4065, 1.7001)
  line L104 (-5.889, -3.4) -> (-5.371, -1.9923)
  line L105 (-5.889, -3.4) -> (-4.4109, -3.6553)
  line L106 (-5.889, -3.4) -> (-6.4069, -4.8077)
  line L107 (-5.889, -3.4) -> (-7.3671, -3.1447)
  line L108 (6.4069, -4.8077) -> (15.4284, -1.4885)
  line L109 (5.889, -3.4) -> (15.4994, 0.136)
  line L110 (5.371, -1.9923) -> (15.4065, 1.7001)
  line L111 (7.3671, -3.1447) -> (9.0033, -12.6171)
  line L112 (5.889, -3.4) -> (7.632, -13.4909)
  line L113 (4.4109, -3.6553) -> (6.2309, -14.1924)
  line L114 (5.889, -3.4) -> (4.4109, -3.6553)
  line L115 (5.889, -3.4) -> (5.371, -1.9923)
  line L116 (5.889, -3.4) -> (7.3671, -3.1447)
  line L117 (5.889, -3.4) -> (6.4069, -4.8077)
  dimension "d1" = 55
  dimension "d2" = 10.5
  dimension "d3" = 3.3
  dimension "d4" = 6.6
  dimension "d5" = 10.5
  dimension "d7" = 360
  dimension "d8" = 1.5
  dimension "d9" = 4.2
  dimension "d10" = 2.5
  dimension "d11" = 5
  dimension "d12" = 5
  dimension "d13" = 2.1
  dimension "d15" = 360
  dimension "d16" = 6.8
  dimension "d17" = 39.8
  dimension "d18" = 1.5
  dimension "d19" = 1.5
  dimension "d56" = 360
  constraint coincident A0.centre L0.start
  constraint coincident A0 L0.end
  constraint vertical L0
  constraint parallel L0 L1
  constraint perpendicular L0 L2
  constraint coincident A0 L3.end
  constraint perpendicular L2 L3
  constraint horizontal L4
  constraint vertical L5
  constraint horizontal L6
  constraint vertical L7
  constraint perpendicular L2 L63
  constraint concentric A0 A1
  constraint coincident L63.end A1
  constraint coincident L0 L64.start
  constraint coincident A2 L64.start
  constraint perpendicular L0 L64
  constraint coincident A1 L65.end
  constraint perpendicular L64 L65
  constraint horizontal L66
  constraint vertical L67
  constraint horizontal L68
  constraint vertical L69
  constraint coincident A1 L67.end
  constraint horizontal L70
  constraint vertical L71
  constraint horizontal L72
  constraint vertical L73
  constraint parallel L0 L84
  constraint coincident L67 L85.end
  constraint perpendicular L67 L85
  constraint coincident L69 L86.end
  constraint perpendicular L69 L86
  constraint horizontal L88
  constraint coincident A1 L87.end
  constraint perpendicular L87 L89
  constraint coincident A1 L90.end
  constraint perpendicular L89 L90
  constraint perpendicular L87 L91
  constraint coincident A1 L92.end
  constraint perpendicular L91 L92
  constraint symmetric L0 L84.end L85.start
  constraint symmetric L0 L87.end L95.end
  constraint symmetric L0 L89.end L94.start
  constraint symmetric L0 L90.end L94.end
  constraint symmetric L0 L91.end L93.start
  constraint symmetric L0 L92.end L93.end
  measures "d1" diameter of A0
  measures "d2" distance of L0.end L1.end
  measures "d3" distance of L1.end L2.end
  measures "d4" distance of L2.end L4.end
  measures "d5" distance of L2.end L6.end
  measures "d8" distance of L1.end L63.end
  measures "d9" diameter of A2
  measures "d10" distance of L64.start L64.end
  measures "d11" distance of L64.end L66.end
  measures "d12" distance of L66.end L64.end
  measures "d13" distance of L66.end L72.end
  measures "d16" distance of A0.centre L84.end
  measures "d17" angle of L87 L88
  measures "d18" distance of L84.end L89.end
  measures "d19" distance of L84.end L91.end
extrude "押し出し1" add sketch "スケッチ1" along normal blind 1.5 contours A0 L2 L3 L4 L5 L7 L8 L9 L10 L12 L13 L14 L15 L17 L18 L19 L20 L22 L23 L24 L25 L27 L28 L29 L30 L32 L33 L34 L35 L37 L38 L39 L40 L42 L43 L44 L45 L47 L48 L49 L50 L52 L53 L54 L55 L57 L58 L59 L60 L62 | L0 L66 L67 L70 L76 L78 L84 L85 L94 L96 | A2 L64 L66 L70 L83 | L0 L64 L65 L66 L69 L70 L79 L83 L84 L86 L89 L90 | A2 L66 L70 L78 | A2 L71 L72 L74 L78 L79 L80 L81 L82 L110 L113 L114 L115 | A2 L64 L66 L70 L71 L72 L79 L83 | A2 L66 L70 L72 L73 L76 L78 | A2 L72 L73 L74 L75 L76 L77 L81 L83 L100 L103 L104 L105 | A2 L74 L78 L81 L83 | L0 L91 L92 | L85 L94 L96 | L65 L69 L86 L87 L90 | L65 L69 L87 L92 L93 L97 | L86 L89 L90 | L67 L91 L92 L93 L95 | L67 L85 L94 L95 | L0 L93 L97 | L64 L66 L70 L79 L83 | L66 L70 L76 L78 | L67 L85 L94 | L65 L69 L86 L90 | A1 L65 L69 L87 L90 | A1 L65 L69 L87 L92 | A1 L67 L93 L95 | A1 L67 L94 L95 | L64 L66 L70 L71 L79 | L66 L70 L73 L76 | A1 L80 L109 L110 | L80 L109 L110 L115 | L77 L102 L103 L104 | A1 L77 L102 L103 | A1 L75 L99 L100 | L75 L99 L100 L105 | L82 L112 L113 L114 | A1 L82 L112 L113 | A1 L80 L108 L109 | L80 L108 L109 L111 L116 | L77 L98 L101 L102 L107 | A1 L77 L101 L102 | A1 L75 L98 L99 | L75 L98 L99 L101 L106 | L82 L108 L111 L112 L117 | A1 L82 L111 L112 | L108 L111 L116 L117 | L98 L101 L106 L107
sketch "スケッチ2" plane through (0, 0, 1.5) normal (0, 0, 1) x (-1, 0, 0)
  line L0 (-5.6421, -16.3724) -> (-10.7928, -25.2936)
  arc A0 (-10.7928, -25.2936) -> (-3.3, -27.3013) centre (0, 0) ccw
  line L1 (-3.3, -27.3013) -> (-3.3, -17)
  line L2 (-3.3, -17) -> (3.3, -17)
  line L3 (3.3, -17) -> (3.3, -27.3013)
  arc A1 (3.3, -27.3013) -> (10.7928, -25.2936) centre (0, 0) ccw
  line L4 (10.7928, -25.2936) -> (5.6421, -16.3724)
  line L5 (5.6421, -16.3724) -> (11.3579, -13.0724)
  line L6 (11.3579, -13.0724) -> (16.5085, -21.9936)
  arc A2 (16.5085, -21.9936) -> (21.9936, -16.5085) centre (0, 0) ccw
  line L7 (21.9936, -16.5085) -> (13.0724, -11.3579)
  line L8 (13.0724, -11.3579) -> (16.3724, -5.6421)
  line L9 (16.3724, -5.6421) -> (25.2936, -10.7928)
  arc A3 (25.2936, -10.7928) -> (27.3013, -3.3) centre (0, 0) ccw
  line L10 (27.3013, -3.3) -> (17, -3.3)
  line L11 (17, -3.3) -> (17, 3.3)
  line L12 (17, 3.3) -> (27.3013, 3.3)
  arc A4 (27.3013, 3.3) -> (25.2936, 10.7928) centre (0, 0) ccw
  line L13 (25.2936, 10.7928) -> (16.3724, 5.6421)
  line L14 (16.3724, 5.6421) -> (13.0724, 11.3579)
  line L15 (13.0724, 11.3579) -> (21.9936, 16.5085)
  arc A5 (21.9936, 16.5085) -> (16.5085, 21.9936) centre (0, 0) ccw
  line L16 (16.5085, 21.9936) -> (11.3579, 13.0724)
  line L17 (11.3579, 13.0724) -> (5.6421, 16.3724)
  line L18 (5.6421, 16.3724) -> (10.7928, 25.2936)
  arc A6 (10.7928, 25.2936) -> (3.3, 27.3013) centre (0, 0) ccw
  line L19 (3.3, 27.3013) -> (3.3, 17)
  line L20 (3.3, 17) -> (-3.3, 17)
  line L21 (-3.3, 17) -> (-3.3, 27.3013)
  arc A7 (-3.3, 27.3013) -> (-10.7928, 25.2936) centre (0, 0) ccw
  line L22 (-10.7928, 25.2936) -> (-5.6421, 16.3724)
  line L23 (-5.6421, 16.3724) -> (-11.3579, 13.0724)
  line L24 (-11.3579, 13.0724) -> (-16.5085, 21.9936)
  arc A8 (-16.5085, 21.9936) -> (-21.9936, 16.5085) centre (0, 0) ccw
  line L25 (-21.9936, 16.5085) -> (-13.0724, 11.3579)
  line L26 (-13.0724, 11.3579) -> (-16.3724, 5.6421)
  line L27 (-16.3724, 5.6421) -> (-25.2936, 10.7928)
  arc A9 (-25.2936, 10.7928) -> (-27.3013, 3.3) centre (0, 0) ccw
  line L28 (-27.3013, 3.3) -> (-17, 3.3)
  line L29 (-17, 3.3) -> (-17, -3.3)
  line L30 (-17, -3.3) -> (-27.3013, -3.3)
  arc A10 (-27.3013, -3.3) -> (-25.2936, -10.7928) centre (0, 0) ccw
  line L31 (-25.2936, -10.7928) -> (-16.3724, -5.6421)
  line L32 (-16.3724, -5.6421) -> (-13.0724, -11.3579)
  line L33 (-13.0724, -11.3579) -> (-21.9936, -16.5085)
  arc A11 (-21.9936, -16.5085) -> (-16.5085, -21.9936) centre (0, 0) ccw
  line L34 (-16.5085, -21.9936) -> (-11.3579, -13.0724)
  line L35 (-11.3579, -13.0724) -> (-5.6421, -16.3724)
  line L36 (0, 0) -> (0, -6.25)
  circle A12 centre (0, -6.25) radius 2.5
  circle A13 centre (0, -6.25) radius 1.65
  circle A14 centre (5.4127, 3.125) radius 2.5
  circle A15 centre (5.4127, 3.125) radius 1.65
  circle A16 centre (-5.4127, 3.125) radius 2.5
  circle A17 centre (-5.4127, 3.125) radius 1.65
  line L37 (4.752, 5.6303) -> (0, 2.8868)
  line L38 (0, 2.8868) -> (-4.752, 5.6303)
  line L39 (-4.752, 5.6303) -> (-6.2309, 14.1924)
  arc A18 (6.2309, 14.1924) -> (-6.2309, 14.1924) centre (0, 0) ccw
  line L40 (6.2309, 14.1924) -> (4.752, 5.6303)
  circle A19 centre (0, 0) radius 2.1
  arc A20 (15.4284, 1.4885) -> (9.0033, 12.6171) centre (0, 0) ccw
  line L41 (15.4284, 1.4885) -> (7.5798, 4.3762)
  line L42 (7.5798, 4.3762) -> (9.0033, 12.6171)
  line L43 (2.5, -6.9305) -> (2.5, -1.4434)
  line L44 (2.5, -1.4434) -> (7.252, 1.3002)
  line L45 (7.252, 1.3002) -> (15.4065, -1.7001)
  arc A21 (9.1755, -12.4924) -> (15.4065, -1.7001) centre (0, 0) ccw
  line L46 (9.1755, -12.4924) -> (2.5, -6.9305)
  arc A22 (-9.0033, 12.6171) -> (-15.4284, 1.4885) centre (0, 0) ccw
  line L47 (-9.0033, 12.6171) -> (-7.5798, 4.3762)
  line L48 (-7.5798, 4.3762) -> (-15.4284, 1.4885)
  line L49 (-6.4251, -14.1056) -> (0, -8.7524)
  line L50 (0, -8.7524) -> (6.4251, -14.1056)
  arc A23 (-6.4251, -14.1056) -> (6.4251, -14.1056) centre (0, 0) ccw
  line L51 (-2.5, -6.9305) -> (-9.1755, -12.4924)
  arc A24 (-15.4065, -1.7001) -> (-9.1755, -12.4924) centre (0, 0) ccw
  line L52 (-15.4065, -1.7001) -> (-7.252, 1.3002)
  line L53 (-7.252, 1.3002) -> (-2.5, -1.4434)
  line L54 (-2.5, -1.4434) -> (-2.5, -6.9305)
  dimension "d25" = 6.25
  dimension "d26" = 5
  dimension "d27" = 3.3
  dimension "d29" = 360
  constraint coincident A0.centre A1.centre
  constraint vertical L36
  constraint coincident L36.end A12.centre
  constraint concentric A12 A13
  measures "d25" distance of A0.centre L36.end
  measures "d26" diameter of A12
  measures "d27" diameter of A13
extrude "押し出し2" cut sketch "スケッチ2" against normal blind 1.5 contours A13 | A15 | A17